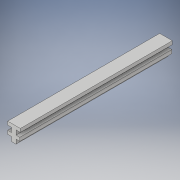
# Autodesk Inventor part: RIPnewslide2
Saved by Autodesk Inventor 2017 (Build 210142000, 142)
## iProperties
Created: 2017-11-22
Part Number: RIPnewslide2
Material: Generic
Document SubType Name: Modeling
Designer: build
Density: 1 g/cm^3
Appearance: Default
Author: build
Autodesk Inventor part; units mm, degrees
ref_plane "YZ Plane" through (0, 0, 0) normal (1, 0, 0) x (0, 1, 0)
ref_plane "XZ Plane" through (0, 0, 0) normal (0, 1, 0) x (-1, 0, 0)
ref_plane "XY Plane" through (0, 0, 0) normal (0, 0, 1) x (1, 0, 0)
sketch "Sketch1" plane through (0, 0, 0) normal (0, 0, 1) x (1, 0, 0)
  point P0 (0, 0)
sketch "Sketch2" plane through (0, 0, 0) normal (0, 0, 1) x (1, 0, 0)
  point P0 (0, 0)
sketch "Sketch3" plane through (0, 0, 0) normal (0, 0, 1) x (1, 0, 0)
  line L0 (7.62, 10.922) -> (7.62, 14.351)
  line L1 (7.62, 14.351) -> (-5.08, 14.351)
  line L2 (-5.08, 14.351) -> (-5.08, 10.922)
  line L3 (-5.08, 10.922) -> (-1.27, 10.922)
  line L4 (-1.27, 10.922) -> (-1.27, 6.477)
  line L5 (-1.27, 6.477) -> (-5.08, 6.477)
  line L6 (-5.08, 6.477) -> (-5.08, 2.921)
  line L7 (-5.08, 2.921) -> (-1.27, 2.921)
  line L8 (-1.27, 2.921) -> (-1.27, -1.397)
  line L9 (-1.27, -1.397) -> (3.302, -1.397)
  line L10 (3.302, -1.397) -> (3.302, 2.921)
  line L11 (3.302, 2.921) -> (7.112, 2.921)
  line L12 (7.112, 2.921) -> (7.112, 6.477)
  line L13 (7.112, 6.477) -> (3.302, 6.477)
  line L14 (3.302, 6.477) -> (3.302, 10.922)
  line L15 (3.302, 10.922) -> (7.62, 10.922)
  point P0 (0, 0)
  dimension "d6" = 3.429
  dimension "d7" = 12.7
  dimension "d9" = 3.429
  dimension "d12" = 3.81
  dimension "d13" = 4.445
  dimension "d14" = 3.556
  dimension "d15" = 4.572
  dimension "d16" = 4.318
  dimension "d17" = 3.556
  dimension "d21" = 4.318
  constraints: 32 end point, 10 perpendicular, 4 point on line, 2 vertical, 1 horizontal
  measures "d6" distance of L0.start L0.end
  measures "d7" distance of L0.end L1.end
  measures "d9" distance of L1.end L2.end
  measures "d12" distance of L2.end L3.end
  measures "d13" distance of L3.end L4.end
  measures "d14" distance of L5.end L6.end
  measures "d15" distance of L8.end L9.end
  measures "d16" distance of L7.end L8.end
  measures "d17" distance of L11.end L12.end
  measures "d21" distance of L9.end L10.end
extrude "Extrusion1" add sketch "Sketch3" along normal blind 152.4
shell "Shell1" thickness 1.27 removed faces 0
body "Solid1"
